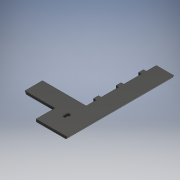
# Autodesk Inventor part: BA10
Saved by Autodesk Inventor 2017 (Build 210142000, 142)
## iProperties
Created: 2019-05-29
Part Number: BA10
Material: Wood (Cherry)
Document SubType Name: Modeling
Designer: Dell
Density: 0.63 g/cm^3
Appearance: Smooth - Black
Author: Dell
Autodesk Inventor part; units mm, degrees
ref_plane "YZ Plane" through (0, 0, 0) normal (1, 0, 0) x (0, 1, 0)
ref_plane "XZ Plane" through (0, 0, 0) normal (0, 1, 0) x (-1, 0, 0)
ref_plane "XY Plane" through (0, 0, 0) normal (0, 0, 1) x (1, 0, 0)
sketch "Sketch1" plane through (0, 0, 0) normal (0, 0, 1) x (1, 0, 0)
  line L0 (0, 0) -> (0, 355.6)
  line L1 (0, 355.6) -> (88.9, 355.6)
  line L2 (88.9, 355.6) -> (88.9, -184.15)
  line L3 (88.9, -184.15) -> (-221.9917, -184.15) construction
  line L4 (-221.9917, -184.15) -> (-221.9917, 0) construction
  line L5 (-221.9917, 0) -> (0, 0)
  line L6 (-221.9917, -184.15) -> (-69.5917, -184.15) construction
  line L7 (-69.5917, -184.15) -> (-69.5917, -88.9)
  line L8 (-69.5917, -88.9) -> (-221.9917, -88.9)
  line L9 (-221.9917, -88.9) -> (-221.9917, -184.15) construction
  line L10 (-221.9917, -88.9) -> (-221.9917, 0)
  line L11 (-69.5917, -184.15) -> (88.9, -184.15)
  line L12 (0, 304.8) -> (-13.97, 304.8)
  line L13 (-13.97, 304.8) -> (-13.97, 279.4)
  line L14 (-13.97, 279.4) -> (0, 279.4)
  line L15 (0, 279.4) -> (0, 304.8)
  line L16 (0, 165.1) -> (-13.97, 165.1)
  line L17 (-13.97, 165.1) -> (-13.97, 190.5)
  line L18 (-13.97, 190.5) -> (0, 190.5)
  line L19 (0, 190.5) -> (0, 165.1)
  line L20 (0, 76.2) -> (-13.97, 76.2)
  line L21 (-13.97, 76.2) -> (-13.97, 50.8)
  line L22 (-13.97, 50.8) -> (0, 50.8)
  line L23 (0, 50.8) -> (0, 76.2)
  line L24 (-12.7, -79.375) -> (0, -79.375)
  line L25 (0, -79.375) -> (0, -104.775)
  line L26 (0, -104.775) -> (-12.7, -104.775)
  line L27 (-12.7, -104.775) -> (-12.7, -79.375)
  line L28 (-13.97, -78.105) -> (1.27, -78.105)
  line L29 (1.27, -78.105) -> (1.27, -106.045)
  line L30 (1.27, -106.045) -> (-13.97, -106.045)
  line L31 (-13.97, -106.045) -> (-13.97, -78.105)
  point P0 (0, 177.8)
  point P1 (0, -92.075)
  point P2 (-12.7, -92.075)
  point P3 (-13.97, -92.075)
  point P4 (-6.35, -79.375)
  point P5 (-6.35, -78.105)
  point P6 (-221.9917, -92.075)
  dimension "d0" = 88.9
  dimension "d1" = 355.6
  dimension "d2" = 310.8917
  dimension "d3" = 184.15
  dimension "d4" = 152.4
  dimension "d5" = 95.25
  dimension "d6" = 13.97
  dimension "d7" = 25.4
  dimension "d8" = 25.4
  dimension "d9" = 25.4
  dimension "d10" = 50.8
  dimension "d11" = 50.8
  dimension "d12" = 12.7
  dimension "d13" = 25.4
  dimension "d14" = 1.27
  dimension "d15" = 1.27
  constraints: 64 end point, 12 parallel, 10 perpendicular, 8 midpoint, 7 horizontal, 4 point on line, 3 vertical alignment, 2 horizontal alignment, 2 vertical, 1 collinear
  measures "d0" distance between parallel lines of L2 L0
  measures "d1" distance of L0.start L0.end
  measures "d2" distance between parallel lines of L4 L2
  measures "d3" distance of L3.end L4.end
  measures "d4" distance of L7.end L8.end
  measures "d5" distance of L6.end L7.end
  measures "d6" distance of L14.end L13.end
  measures "d7" distance of L12.end L13.end
  measures "d8" distance of L16.end L17.end
  measures "d9" distance of L20.end L21.end
  measures "d10" distance between parallel lines of L1 L12
  measures "d11" distance between parallel lines of L5 L22
  measures "d12" distance of L25.end L26.end
  measures "d13" distance of L24.end L25.end
  measures "d14" distance between parallel lines of L28 L24
  measures "d15" distance between parallel lines of L29 L25
extrude "Extrusion1" add sketch "Sketch1" along normal blind 12.7 contours L0 L1 L2 L11 L7 L8 L10 L5 | L22 L21 L20 L0 | L16 L17 L18 L0 | L14 L13 L12 L0
sketch "Sketch3" plane through (0, 355.6, 0) normal (0, 1, 0) x (1, 0, 0)
  line L0 (88.9, -12.7) -> (81.5677, 0)
  line L1 (-69.5917, 0) -> (88.9, 0) projected
  line L2 (88.9, 0) -> (81.5677, 0)
  line L3 (88.9, 0) -> (88.9, -12.7)
  line L4 (-221.9917, -12.7) -> (-214.6593, 0)
  line L5 (0, 0) -> (-221.9917, 0) projected
  line L6 (-214.6593, 0) -> (-221.9917, 0)
  line L7 (-221.9917, 0) -> (-221.9917, -12.7) projected
  line L8 (-221.9917, 0) -> (-221.9917, -12.7)
  dimension "d18" = 30
  dimension "d19" = 30
  constraints: 12 end point, 2 collinear, 2 perpendicular, 1 point on line
  measures "d18" angle of L3 L0
  measures "d19" angle of L7 L4
extrude "Extrusion2" cut sketch "Sketch3" against normal through all
body "Solid1"
